Autodesk Fusion 360 part; units mm, degrees
note: some values were not read from the file. Chosen so that the rebuilt part matches the saved one: which bodies a step acts on; a direction. Set by a fixed rule: which sketch regions a step uses.
(part 3 of 5)
extrude "VL53L0X chip FL" add sketch "VL53L0X chip FL sketch" along normal blind 2.4 from surface at 101.6 separate body makes body 56 in component "ToF FL"
sketch "M2.5 screw heads FL sketch" plane through (0, 0, 0) normal (0, 0, 1) x (1, 0, 0) in component "ToF FL"
  line L0 (84.9852, 42.2659) -> (86.3446, 42.8999)
  line L1 (86.3446, 42.8999) -> (84.4428, 46.9782)
  line L2 (84.4428, 46.9782) -> (83.0834, 46.3443)
  line L3 (83.0834, 46.3443) -> (84.9852, 42.2659)
  line L4 (90.3524, 30.7558) -> (91.7119, 31.3898)
  line L5 (91.7119, 31.3898) -> (89.8101, 35.4681)
  line L6 (89.8101, 35.4681) -> (88.4506, 34.8342)
  line L7 (88.4506, 34.8342) -> (90.3524, 30.7558)
extrude "M2.5 screw heads FL" add sketch "M2.5 screw heads FL sketch" along normal blind 4.5 from surface at 110.71 separate body makes body 57 at (84.3512, 43.6254, 113.71) makes body 58 at (89.0846, 33.4748, 112.21) in component "ToF FL"
sketch "M2.5 screw shafts FL sketch" plane through (0, 0, 0) normal (0, 0, 1) x (1, 0, 0) in component "ToF FL"
  line L0 (85.8164, 44.0327) -> (91.2542, 46.5685)
  line L1 (91.2542, 46.5685) -> (90.409, 48.3811)
  line L2 (90.409, 48.3811) -> (84.9711, 45.8454)
  line L3 (84.9711, 45.8454) -> (85.8164, 44.0327)
  line L4 (91.1836, 32.5226) -> (96.6215, 35.0583)
  line L5 (96.6215, 35.0583) -> (95.7762, 36.871)
  line L6 (95.7762, 36.871) -> (90.3384, 34.3353)
  line L7 (90.3384, 34.3353) -> (91.1836, 32.5226)
extrude "M2.5 screw shafts FL" add sketch "M2.5 screw shafts FL sketch" along normal blind 2 from surface at 111.96 separate body makes body 59 at (88.8781, 46.9316, 111.96) makes body 60 at (93.9636, 36.0257, 112.6267) in component "ToF FL"
sketch "VL53L0X board FR sketch" plane through (0, 0, 0) normal (0, 0, 1) x (1, 0, 0) in component "ToF FR"
  line L0 (84.3203, -47.2411) -> (85.7704, -47.9173)
  line L1 (85.7704, -47.9173) -> (93.2845, -31.8031)
  line L2 (93.2845, -31.8031) -> (91.8344, -31.1269)
  line L3 (91.8344, -31.1269) -> (84.3203, -47.2411)
extrude "VL53L0X board FR" add sketch "VL53L0X board FR sketch" along normal blind 25.4 from surface at 90.1 separate body makes body 61 in component "ToF FR"
sketch "Board holes sketch (3)" plane through (0, 0, 0) normal (0, 0, 1) x (1, 0, 0) in component "ToF FR"
  line L0 (89.7796, -34.3505) -> (92.136, -35.4493)
  line L1 (92.136, -35.4493) -> (93.1925, -33.1836)
  line L2 (93.1925, -33.1836) -> (90.8361, -32.0848)
  line L3 (90.8361, -32.0848) -> (89.7796, -34.3505)
  line L4 (84.4123, -45.8606) -> (86.7687, -46.9594)
  line L5 (86.7687, -46.9594) -> (87.8253, -44.6937)
  line L6 (87.8253, -44.6937) -> (85.4689, -43.5949)
  line L7 (85.4689, -43.5949) -> (84.4123, -45.8606)
extrude "Board holes''" cut sketch "Board holes sketch (3)" along normal blind 2.5 from surface at 111.71 bodies 61 in component "ToF FR"
sketch "Board holes sketch (1) (3)" plane through (0, 0, 0) normal (0, 0, 1) x (1, 0, 0) in component "ToF FR"
  line L0 (89.7796, -34.3505) -> (92.136, -35.4493)
  line L1 (92.136, -35.4493) -> (93.1925, -33.1836)
  line L2 (93.1925, -33.1836) -> (90.8361, -32.0848)
  line L3 (90.8361, -32.0848) -> (89.7796, -34.3505)
  line L4 (84.4123, -45.8606) -> (86.7687, -46.9594)
  line L5 (86.7687, -46.9594) -> (87.8253, -44.6937)
  line L6 (87.8253, -44.6937) -> (85.4689, -43.5949)
  line L7 (85.4689, -43.5949) -> (84.4123, -45.8606)
extrude "Board holes (1)''" cut sketch "Board holes sketch (1) (3)" along normal blind 2.5 from surface at 91.39 bodies 61 in component "ToF FR"
sketch "QT connector FR sketch" plane through (0, 0, 0) normal (0, 0, 1) x (1, 0, 0) in component "ToF FR"
  line L0 (88.2385, -42.6244) -> (91.0027, -43.9134)
  line L1 (91.0027, -43.9134) -> (93.5807, -38.3849)
  line L2 (93.5807, -38.3849) -> (90.8164, -37.096)
  line L3 (90.8164, -37.096) -> (88.2385, -42.6244)
extrude "QT connector FR" add sketch "QT connector FR sketch" along normal blind 4.25 from surface at 110.67 separate body makes body 62 in component "ToF FR"
sketch "QT connector FR sketch (1)" plane through (0, 0, 0) normal (0, 0, 1) x (1, 0, 0) in component "ToF FR"
  line L0 (88.2385, -42.6244) -> (91.0027, -43.9134)
  line L1 (91.0027, -43.9134) -> (93.5807, -38.3849)
  line L2 (93.5807, -38.3849) -> (90.8164, -37.096)
  line L3 (90.8164, -37.096) -> (88.2385, -42.6244)
extrude "QT connector FR (1)" add sketch "QT connector FR sketch (1)" along normal blind 4.25 from surface at 90.68 separate body makes body 63 in component "ToF FR"
sketch "VL53L0X chip FR sketch" plane through (0, 0, 0) normal (0, 0, 1) x (1, 0, 0) in component "ToF FR"
  line L0 (88.5977, -41.8541) -> (89.504, -42.2767)
  line L1 (89.504, -42.2767) -> (91.3635, -38.2889)
  line L2 (91.3635, -38.2889) -> (90.4572, -37.8663)
  line L3 (90.4572, -37.8663) -> (88.5977, -41.8541)
extrude "VL53L0X chip FR" add sketch "VL53L0X chip FR sketch" along normal blind 2.4 from surface at 101.6 separate body makes body 64 in component "ToF FR"
sketch "M2.5 screw heads FR sketch" plane through (0, 0, 0) normal (0, 0, 1) x (1, 0, 0) in component "ToF FR"
  line L0 (88.4506, -34.8342) -> (89.8101, -35.4681)
  line L1 (89.8101, -35.4681) -> (91.7119, -31.3898)
  line L2 (91.7119, -31.3898) -> (90.3524, -30.7558)
  line L3 (90.3524, -30.7558) -> (88.4506, -34.8342)
  line L4 (83.0834, -46.3443) -> (84.4428, -46.9782)
  line L5 (84.4428, -46.9782) -> (86.3446, -42.8999)
  line L6 (86.3446, -42.8999) -> (84.9852, -42.2659)
  line L7 (84.9852, -42.2659) -> (83.0834, -46.3443)
extrude "M2.5 screw heads FR" add sketch "M2.5 screw heads FR sketch" along normal blind 4.5 from surface at 110.71 separate body makes body 65 at (89.7185, -32.1153, 112.21) makes body 66 at (83.7173, -44.9849, 113.71) in component "ToF FR"
sketch "M2.5 screw shafts FR sketch" plane through (0, 0, 0) normal (0, 0, 1) x (1, 0, 0) in component "ToF FR"
  line L0 (90.3384, -34.3353) -> (95.7762, -36.871)
  line L1 (95.7762, -36.871) -> (96.6215, -35.0583)
  line L2 (96.6215, -35.0583) -> (91.1836, -32.5226)
  line L3 (91.1836, -32.5226) -> (90.3384, -34.3353)
  line L4 (84.9711, -45.8454) -> (90.409, -48.3811)
  line L5 (90.409, -48.3811) -> (91.2542, -46.5685)
  line L6 (91.2542, -46.5685) -> (85.8164, -44.0327)
  line L7 (85.8164, -44.0327) -> (84.9711, -45.8454)
extrude "M2.5 screw shafts FR" add sketch "M2.5 screw shafts FR sketch" along normal blind 2 from surface at 111.96 separate body makes body 67 at (94.8088, -34.2131, 112.6267) makes body 68 at (87.3472, -45.4822, 111.96) in component "ToF FR"
sketch "VL53L0X board SFL sketch" plane through (0, 0, 0) normal (0, 0, 1) x (1, 0, 0) in component "ToF SFL"
  line L0 (77.39, 58.4) -> (77.39, 60)
  line L1 (77.39, 60) -> (59.61, 60)
  line L2 (59.61, 60) -> (59.61, 58.4)
  line L3 (59.61, 58.4) -> (77.39, 58.4)
extrude "VL53L0X board SFL" add sketch "VL53L0X board SFL sketch" along normal blind 25.4 from surface at 90.1 separate body makes body 69 in component "ToF SFL"
sketch "Board holes sketch (4)" plane through (0, 0, 0) normal (0, 0, 1) x (1, 0, 0) in component "ToF SFL"
  line L0 (63.4, 57.9) -> (63.4, 60.5)
  line L1 (63.4, 60.5) -> (60.9, 60.5)
  line L2 (60.9, 60.5) -> (60.9, 57.9)
  line L3 (60.9, 57.9) -> (63.4, 57.9)
  line L4 (76.1, 57.9) -> (76.1, 60.5)
  line L5 (76.1, 60.5) -> (73.6, 60.5)
  line L6 (73.6, 60.5) -> (73.6, 57.9)
  line L7 (73.6, 57.9) -> (76.1, 57.9)
extrude "Board holes'''" cut sketch "Board holes sketch (4)" along normal blind 2.5 from surface at 111.71 bodies 69 in component "ToF SFL"
sketch "Board holes sketch (1) (4)" plane through (0, 0, 0) normal (0, 0, 1) x (1, 0, 0) in component "ToF SFL"
  line L0 (63.4, 57.9) -> (63.4, 60.5)
  line L1 (63.4, 60.5) -> (60.9, 60.5)
  line L2 (60.9, 60.5) -> (60.9, 57.9)
  line L3 (60.9, 57.9) -> (63.4, 57.9)
  line L4 (76.1, 57.9) -> (76.1, 60.5)
  line L5 (76.1, 60.5) -> (73.6, 60.5)
  line L6 (73.6, 60.5) -> (73.6, 57.9)
  line L7 (73.6, 57.9) -> (76.1, 57.9)
extrude "Board holes (1)'''" cut sketch "Board holes sketch (1) (4)" along normal blind 2.5 from surface at 91.39 bodies 69 in component "ToF SFL"
sketch "QT connector SFL sketch" plane through (0, 0, 0) normal (0, 0, 1) x (1, 0, 0) in component "ToF SFL"
  line L0 (71.55, 60) -> (71.55, 63.05)
  line L1 (71.55, 63.05) -> (65.45, 63.05)
  line L2 (65.45, 63.05) -> (65.45, 60)
  line L3 (65.45, 60) -> (71.55, 60)
extrude "QT connector SFL" add sketch "QT connector SFL sketch" along normal blind 4.25 from surface at 110.67 separate body makes body 70 in component "ToF SFL"
sketch "QT connector SFL sketch (1)" plane through (0, 0, 0) normal (0, 0, 1) x (1, 0, 0) in component "ToF SFL"
  line L0 (71.55, 60) -> (71.55, 63.05)
  line L1 (71.55, 63.05) -> (65.45, 63.05)
  line L2 (65.45, 63.05) -> (65.45, 60)
  line L3 (65.45, 60) -> (71.55, 60)
extrude "QT connector SFL (1)" add sketch "QT connector SFL sketch (1)" along normal blind 4.25 from surface at 90.68 separate body makes body 71 in component "ToF SFL"
sketch "VL53L0X chip SFL sketch" plane through (0, 0, 0) normal (0, 0, 1) x (1, 0, 0) in component "ToF SFL"
  line L0 (70.7, 60) -> (70.7, 61)
  line L1 (70.7, 61) -> (66.3, 61)
  line L2 (66.3, 61) -> (66.3, 60)
  line L3 (66.3, 60) -> (70.7, 60)
extrude "VL53L0X chip SFL" add sketch "VL53L0X chip SFL sketch" along normal blind 2.4 from surface at 101.6 separate body makes body 72 in component "ToF SFL"
sketch "M2.5 screw heads SFL sketch" plane through (0, 0, 0) normal (0, 0, 1) x (1, 0, 0) in component "ToF SFL"
  line L0 (64.4, 56.9) -> (64.4, 58.4)
  line L1 (64.4, 58.4) -> (59.9, 58.4)
  line L2 (59.9, 58.4) -> (59.9, 56.9)
  line L3 (59.9, 56.9) -> (64.4, 56.9)
  line L4 (77.1, 56.9) -> (77.1, 58.4)
  line L5 (77.1, 58.4) -> (72.6, 58.4)
  line L6 (72.6, 58.4) -> (72.6, 56.9)
  line L7 (72.6, 56.9) -> (77.1, 56.9)
extrude "M2.5 screw heads SFL" add sketch "M2.5 screw heads SFL sketch" along normal blind 4.5 from surface at 110.71 separate body makes body 73 at (61.4, 56.9, 112.21) makes body 74 at (74.1, 56.9, 112.21) in component "ToF SFL"
sketch "M2.5 screw shafts SFL sketch" plane through (0, 0, 0) normal (0, 0, 1) x (1, 0, 0) in component "ToF SFL"
  line L0 (63.15, 58.4) -> (63.15, 64.4)
  line L1 (63.15, 64.4) -> (61.15, 64.4)
  line L2 (61.15, 64.4) -> (61.15, 58.4)
  line L3 (61.15, 58.4) -> (63.15, 58.4)
  line L4 (75.85, 58.4) -> (75.85, 64.4)
  line L5 (75.85, 64.4) -> (73.85, 64.4)
  line L6 (73.85, 64.4) -> (73.85, 58.4)
  line L7 (73.85, 58.4) -> (75.85, 58.4)
extrude "M2.5 screw shafts SFL" add sketch "M2.5 screw shafts SFL sketch" along normal blind 2 from surface at 111.96 separate body makes body 75 at (61.15, 62.4, 112.6267) makes body 76 at (73.85, 62.4, 112.6267) in component "ToF SFL"
sketch "VL53L0X board SFR sketch" plane through (0, 0, 0) normal (0, 0, 1) x (1, 0, 0) in component "ToF SFR"
  line L0 (59.61, -58.4) -> (59.61, -60)
  line L1 (59.61, -60) -> (77.39, -60)
  line L2 (77.39, -60) -> (77.39, -58.4)
  line L3 (77.39, -58.4) -> (59.61, -58.4)
extrude "VL53L0X board SFR" add sketch "VL53L0X board SFR sketch" along normal blind 25.4 from surface at 90.1 separate body makes body 77 in component "ToF SFR"
sketch "Board holes sketch (5)" plane through (0, 0, 0) normal (0, 0, 1) x (1, 0, 0) in component "ToF SFR"
  line L0 (73.6, -57.9) -> (73.6, -60.5)
  line L1 (73.6, -60.5) -> (76.1, -60.5)
  line L2 (76.1, -60.5) -> (76.1, -57.9)
  line L3 (76.1, -57.9) -> (73.6, -57.9)
  line L4 (60.9, -57.9) -> (60.9, -60.5)
  line L5 (60.9, -60.5) -> (63.4, -60.5)
  line L6 (63.4, -60.5) -> (63.4, -57.9)
  line L7 (63.4, -57.9) -> (60.9, -57.9)
extrude "Board holes''''" cut sketch "Board holes sketch (5)" along normal blind 2.5 from surface at 111.71 bodies 77 in component "ToF SFR"
sketch "Board holes sketch (1) (5)" plane through (0, 0, 0) normal (0, 0, 1) x (1, 0, 0) in component "ToF SFR"
  line L0 (73.6, -57.9) -> (73.6, -60.5)
  line L1 (73.6, -60.5) -> (76.1, -60.5)
  line L2 (76.1, -60.5) -> (76.1, -57.9)
  line L3 (76.1, -57.9) -> (73.6, -57.9)
  line L4 (60.9, -57.9) -> (60.9, -60.5)
  line L5 (60.9, -60.5) -> (63.4, -60.5)
  line L6 (63.4, -60.5) -> (63.4, -57.9)
  line L7 (63.4, -57.9) -> (60.9, -57.9)
extrude "Board holes (1)''''" cut sketch "Board holes sketch (1) (5)" along normal blind 2.5 from surface at 91.39 bodies 77 in component "ToF SFR"
sketch "QT connector SFR sketch" plane through (0, 0, 0) normal (0, 0, 1) x (1, 0, 0) in component "ToF SFR"
  line L0 (65.45, -60) -> (65.45, -63.05)
  line L1 (65.45, -63.05) -> (71.55, -63.05)
  line L2 (71.55, -63.05) -> (71.55, -60)
  line L3 (71.55, -60) -> (65.45, -60)
extrude "QT connector SFR" add sketch "QT connector SFR sketch" along normal blind 4.25 from surface at 110.67 separate body makes body 78 in component "ToF SFR"
sketch "QT connector SFR sketch (1)" plane through (0, 0, 0) normal (0, 0, 1) x (1, 0, 0) in component "ToF SFR"
  line L0 (65.45, -60) -> (65.45, -63.05)
  line L1 (65.45, -63.05) -> (71.55, -63.05)
  line L2 (71.55, -63.05) -> (71.55, -60)
  line L3 (71.55, -60) -> (65.45, -60)
extrude "QT connector SFR (1)" add sketch "QT connector SFR sketch (1)" along normal blind 4.25 from surface at 90.68 separate body makes body 79 in component "ToF SFR"
sketch "VL53L0X chip SFR sketch" plane through (0, 0, 0) normal (0, 0, 1) x (1, 0, 0) in component "ToF SFR"
  line L0 (66.3, -60) -> (66.3, -61)
  line L1 (66.3, -61) -> (70.7, -61)
  line L2 (70.7, -61) -> (70.7, -60)
  line L3 (70.7, -60) -> (66.3, -60)
extrude "VL53L0X chip SFR" add sketch "VL53L0X chip SFR sketch" along normal blind 2.4 from surface at 101.6 separate body makes body 80 in component "ToF SFR"
sketch "M2.5 screw heads SFR sketch" plane through (0, 0, 0) normal (0, 0, 1) x (1, 0, 0) in component "ToF SFR"
  line L0 (72.6, -56.9) -> (72.6, -58.4)
  line L1 (72.6, -58.4) -> (77.1, -58.4)
  line L2 (77.1, -58.4) -> (77.1, -56.9)
  line L3 (77.1, -56.9) -> (72.6, -56.9)
  line L4 (59.9, -56.9) -> (59.9, -58.4)
  line L5 (59.9, -58.4) -> (64.4, -58.4)
  line L6 (64.4, -58.4) -> (64.4, -56.9)
  line L7 (64.4, -56.9) -> (59.9, -56.9)
extrude "M2.5 screw heads SFR" add sketch "M2.5 screw heads SFR sketch" along normal blind 4.5 from surface at 110.71 separate body makes body 81 at (75.6, -56.9, 112.21) makes body 82 at (62.9, -56.9, 112.21) in component "ToF SFR"
sketch "M2.5 screw shafts SFR sketch" plane through (0, 0, 0) normal (0, 0, 1) x (1, 0, 0) in component "ToF SFR"
  line L0 (73.85, -58.4) -> (73.85, -64.4)
  line L1 (73.85, -64.4) -> (75.85, -64.4)
  line L2 (75.85, -64.4) -> (75.85, -58.4)
  line L3 (75.85, -58.4) -> (73.85, -58.4)
  line L4 (61.15, -58.4) -> (61.15, -64.4)
  line L5 (61.15, -64.4) -> (63.15, -64.4)
  line L6 (63.15, -64.4) -> (63.15, -58.4)
  line L7 (63.15, -58.4) -> (61.15, -58.4)
extrude "M2.5 screw shafts SFR" add sketch "M2.5 screw shafts SFR sketch" along normal blind 2 from surface at 111.96 separate body makes body 83 at (75.85, -62.4, 112.6267) makes body 84 at (63.15, -62.4, 112.6267) in component "ToF SFR"
sketch "VL53L0X board SRL sketch" plane through (0, 0, 0) normal (0, 0, 1) x (1, 0, 0) in component "ToF SRL"
  line L0 (-59.61, 58.4) -> (-59.61, 60)
  line L1 (-59.61, 60) -> (-77.39, 60)
  line L2 (-77.39, 60) -> (-77.39, 58.4)
  line L3 (-77.39, 58.4) -> (-59.61, 58.4)
extrude "VL53L0X board SRL" add sketch "VL53L0X board SRL sketch" along normal blind 25.4 from surface at 90.1 separate body makes body 85 in component "ToF SRL"
sketch "Board holes sketch (6)" plane through (0, 0, 0) normal (0, 0, 1) x (1, 0, 0) in component "ToF SRL"
  line L0 (-73.6, 57.9) -> (-73.6, 60.5)
  line L1 (-73.6, 60.5) -> (-76.1, 60.5)
  line L2 (-76.1, 60.5) -> (-76.1, 57.9)
  line L3 (-76.1, 57.9) -> (-73.6, 57.9)
  line L4 (-60.9, 57.9) -> (-60.9, 60.5)
  line L5 (-60.9, 60.5) -> (-63.4, 60.5)
  line L6 (-63.4, 60.5) -> (-63.4, 57.9)
  line L7 (-63.4, 57.9) -> (-60.9, 57.9)
extrude "Board holes'''''" cut sketch "Board holes sketch (6)" along normal blind 2.5 from surface at 111.71 bodies 85 in component "ToF SRL"
sketch "Board holes sketch (1) (6)" plane through (0, 0, 0) normal (0, 0, 1) x (1, 0, 0) in component "ToF SRL"
  line L0 (-73.6, 57.9) -> (-73.6, 60.5)
  line L1 (-73.6, 60.5) -> (-76.1, 60.5)
  line L2 (-76.1, 60.5) -> (-76.1, 57.9)
  line L3 (-76.1, 57.9) -> (-73.6, 57.9)
  line L4 (-60.9, 57.9) -> (-60.9, 60.5)
  line L5 (-60.9, 60.5) -> (-63.4, 60.5)
  line L6 (-63.4, 60.5) -> (-63.4, 57.9)
  line L7 (-63.4, 57.9) -> (-60.9, 57.9)
extrude "Board holes (1)'''''" cut sketch "Board holes sketch (1) (6)" along normal blind 2.5 from surface at 91.39 bodies 85 in component "ToF SRL"
sketch "QT connector SRL sketch" plane through (0, 0, 0) normal (0, 0, 1) x (1, 0, 0) in component "ToF SRL"
  line L0 (-65.45, 60) -> (-65.45, 63.05)
  line L1 (-65.45, 63.05) -> (-71.55, 63.05)
  line L2 (-71.55, 63.05) -> (-71.55, 60)
  line L3 (-71.55, 60) -> (-65.45, 60)
extrude "QT connector SRL" add sketch "QT connector SRL sketch" along normal blind 4.25 from surface at 110.67 separate body makes body 86 in component "ToF SRL"
sketch "QT connector SRL sketch (1)" plane through (0, 0, 0) normal (0, 0, 1) x (1, 0, 0) in component "ToF SRL"
  line L0 (-65.45, 60) -> (-65.45, 63.05)
  line L1 (-65.45, 63.05) -> (-71.55, 63.05)
  line L2 (-71.55, 63.05) -> (-71.55, 60)
  line L3 (-71.55, 60) -> (-65.45, 60)
extrude "QT connector SRL (1)" add sketch "QT connector SRL sketch (1)" along normal blind 4.25 from surface at 90.68 separate body makes body 87 in component "ToF SRL"
sketch "VL53L0X chip SRL sketch" plane through (0, 0, 0) normal (0, 0, 1) x (1, 0, 0) in component "ToF SRL"
  line L0 (-66.3, 60) -> (-66.3, 61)
  line L1 (-66.3, 61) -> (-70.7, 61)
  line L2 (-70.7, 61) -> (-70.7, 60)
  line L3 (-70.7, 60) -> (-66.3, 60)
extrude "VL53L0X chip SRL" add sketch "VL53L0X chip SRL sketch" along normal blind 2.4 from surface at 101.6 separate body makes body 88 in component "ToF SRL"
sketch "M2.5 screw heads SRL sketch" plane through (0, 0, 0) normal (0, 0, 1) x (1, 0, 0) in component "ToF SRL"
  line L0 (-72.6, 56.9) -> (-72.6, 58.4)
  line L1 (-72.6, 58.4) -> (-77.1, 58.4)
  line L2 (-77.1, 58.4) -> (-77.1, 56.9)
  line L3 (-77.1, 56.9) -> (-72.6, 56.9)
  line L4 (-59.9, 56.9) -> (-59.9, 58.4)
  line L5 (-59.9, 58.4) -> (-64.4, 58.4)
  line L6 (-64.4, 58.4) -> (-64.4, 56.9)
  line L7 (-64.4, 56.9) -> (-59.9, 56.9)
extrude "M2.5 screw heads SRL" add sketch "M2.5 screw heads SRL sketch" along normal blind 4.5 from surface at 110.71 separate body makes body 89 at (-75.6, 56.9, 112.21) makes body 90 at (-62.9, 56.9, 112.21) in component "ToF SRL"
sketch "M2.5 screw shafts SRL sketch" plane through (0, 0, 0) normal (0, 0, 1) x (1, 0, 0) in component "ToF SRL"
  line L0 (-73.85, 58.4) -> (-73.85, 64.4)
  line L1 (-73.85, 64.4) -> (-75.85, 64.4)
  line L2 (-75.85, 64.4) -> (-75.85, 58.4)
  line L3 (-75.85, 58.4) -> (-73.85, 58.4)
  line L4 (-61.15, 58.4) -> (-61.15, 64.4)
  line L5 (-61.15, 64.4) -> (-63.15, 64.4)
  line L6 (-63.15, 64.4) -> (-63.15, 58.4)
  line L7 (-63.15, 58.4) -> (-61.15, 58.4)
extrude "M2.5 screw shafts SRL" add sketch "M2.5 screw shafts SRL sketch" along normal blind 2 from surface at 111.96 separate body makes body 91 at (-75.85, 62.4, 112.6267) makes body 92 at (-63.15, 62.4, 112.6267) in component "ToF SRL"
sketch "VL53L0X board SRR sketch" plane through (0, 0, 0) normal (0, 0, 1) x (1, 0, 0) in component "ToF SRR"
  line L0 (-77.39, -58.4) -> (-77.39, -60)
  line L1 (-77.39, -60) -> (-59.61, -60)
  line L2 (-59.61, -60) -> (-59.61, -58.4)
  line L3 (-59.61, -58.4) -> (-77.39, -58.4)
extrude "VL53L0X board SRR" add sketch "VL53L0X board SRR sketch" along normal blind 25.4 from surface at 90.1 separate body makes body 93 in component "ToF SRR"
sketch "Board holes sketch (7)" plane through (0, 0, 0) normal (0, 0, 1) x (1, 0, 0) in component "ToF SRR"
  line L0 (-63.4, -57.9) -> (-63.4, -60.5)
  line L1 (-63.4, -60.5) -> (-60.9, -60.5)
  line L2 (-60.9, -60.5) -> (-60.9, -57.9)
  line L3 (-60.9, -57.9) -> (-63.4, -57.9)
  line L4 (-76.1, -57.9) -> (-76.1, -60.5)
  line L5 (-76.1, -60.5) -> (-73.6, -60.5)
  line L6 (-73.6, -60.5) -> (-73.6, -57.9)
  line L7 (-73.6, -57.9) -> (-76.1, -57.9)
extrude "Board holes''''''" cut sketch "Board holes sketch (7)" along normal blind 2.5 from surface at 111.71 bodies 93 in component "ToF SRR"
sketch "Board holes sketch (1) (7)" plane through (0, 0, 0) normal (0, 0, 1) x (1, 0, 0) in component "ToF SRR"
  line L0 (-63.4, -57.9) -> (-63.4, -60.5)
  line L1 (-63.4, -60.5) -> (-60.9, -60.5)
  line L2 (-60.9, -60.5) -> (-60.9, -57.9)
  line L3 (-60.9, -57.9) -> (-63.4, -57.9)
  line L4 (-76.1, -57.9) -> (-76.1, -60.5)
  line L5 (-76.1, -60.5) -> (-73.6, -60.5)
  line L6 (-73.6, -60.5) -> (-73.6, -57.9)
  line L7 (-73.6, -57.9) -> (-76.1, -57.9)
extrude "Board holes (1)''''''" cut sketch "Board holes sketch (1) (7)" along normal blind 2.5 from surface at 91.39 bodies 93 in component "ToF SRR"
sketch "QT connector SRR sketch" plane through (0, 0, 0) normal (0, 0, 1) x (1, 0, 0) in component "ToF SRR"
  line L0 (-71.55, -60) -> (-71.55, -63.05)
  line L1 (-71.55, -63.05) -> (-65.45, -63.05)
  line L2 (-65.45, -63.05) -> (-65.45, -60)
  line L3 (-65.45, -60) -> (-71.55, -60)
extrude "QT connector SRR" add sketch "QT connector SRR sketch" along normal blind 4.25 from surface at 110.67 separate body makes body 94 in component "ToF SRR"
sketch "QT connector SRR sketch (1)" plane through (0, 0, 0) normal (0, 0, 1) x (1, 0, 0) in component "ToF SRR"
  line L0 (-71.55, -60) -> (-71.55, -63.05)
  line L1 (-71.55, -63.05) -> (-65.45, -63.05)
  line L2 (-65.45, -63.05) -> (-65.45, -60)
  line L3 (-65.45, -60) -> (-71.55, -60)
extrude "QT connector SRR (1)" add sketch "QT connector SRR sketch (1)" along normal blind 4.25 from surface at 90.68 separate body makes body 95 in component "ToF SRR"
sketch "VL53L0X chip SRR sketch" plane through (0, 0, 0) normal (0, 0, 1) x (1, 0, 0) in component "ToF SRR"
  line L0 (-70.7, -60) -> (-70.7, -61)
  line L1 (-70.7, -61) -> (-66.3, -61)
  line L2 (-66.3, -61) -> (-66.3, -60)
  line L3 (-66.3, -60) -> (-70.7, -60)
extrude "VL53L0X chip SRR" add sketch "VL53L0X chip SRR sketch" along normal blind 2.4 from surface at 101.6 separate body makes body 96 in component "ToF SRR"
sketch "M2.5 screw heads SRR sketch" plane through (0, 0, 0) normal (0, 0, 1) x (1, 0, 0) in component "ToF SRR"
  line L0 (-64.4, -56.9) -> (-64.4, -58.4)
  line L1 (-64.4, -58.4) -> (-59.9, -58.4)
  line L2 (-59.9, -58.4) -> (-59.9, -56.9)
  line L3 (-59.9, -56.9) -> (-64.4, -56.9)
  line L4 (-77.1, -56.9) -> (-77.1, -58.4)
  line L5 (-77.1, -58.4) -> (-72.6, -58.4)
  line L6 (-72.6, -58.4) -> (-72.6, -56.9)
  line L7 (-72.6, -56.9) -> (-77.1, -56.9)
extrude "M2.5 screw heads SRR" add sketch "M2.5 screw heads SRR sketch" along normal blind 4.5 from surface at 110.71 separate body makes body 97 at (-61.4, -56.9, 112.21) makes body 98 at (-74.1, -56.9, 112.21) in component "ToF SRR"
sketch "M2.5 screw shafts SRR sketch" plane through (0, 0, 0) normal (0, 0, 1) x (1, 0, 0) in component "ToF SRR"
  line L0 (-63.15, -58.4) -> (-63.15, -64.4)
  line L1 (-63.15, -64.4) -> (-61.15, -64.4)
  line L2 (-61.15, -64.4) -> (-61.15, -58.4)
  line L3 (-61.15, -58.4) -> (-63.15, -58.4)
  line L4 (-75.85, -58.4) -> (-75.85, -64.4)
  line L5 (-75.85, -64.4) -> (-73.85, -64.4)
  line L6 (-73.85, -64.4) -> (-73.85, -58.4)
  line L7 (-73.85, -58.4) -> (-75.85, -58.4)
extrude "M2.5 screw shafts SRR" add sketch "M2.5 screw shafts SRR sketch" along normal blind 2 from surface at 111.96 separate body makes body 99 at (-61.15, -62.4, 112.6267) makes body 100 at (-73.85, -62.4, 112.6267) in component "ToF SRR"
sketch "VL53L0X board RL sketch" plane through (0, 0, 0) normal (0, 0, 1) x (1, 0, 0) in component "ToF RL"
  line L0 (-82.4, 44.89) -> (-84, 44.89)
  line L1 (-84, 44.89) -> (-84, 27.11)
  line L2 (-84, 27.11) -> (-82.4, 27.11)
  line L3 (-82.4, 27.11) -> (-82.4, 44.89)
extrude "VL53L0X board RL" add sketch "VL53L0X board RL sketch" along normal blind 25.4 from surface at 90.1 separate body makes body 101 in component "ToF RL"
sketch "Board holes sketch (8)" plane through (0, 0, 0) normal (0, 0, 1) x (1, 0, 0) in component "ToF RL"
  line L0 (-81.9, 30.9) -> (-84.5, 30.9)
  line L1 (-84.5, 30.9) -> (-84.5, 28.4)
  line L2 (-84.5, 28.4) -> (-81.9, 28.4)
  line L3 (-81.9, 28.4) -> (-81.9, 30.9)
  line L4 (-81.9, 43.6) -> (-84.5, 43.6)
  line L5 (-84.5, 43.6) -> (-84.5, 41.1)
  line L6 (-84.5, 41.1) -> (-81.9, 41.1)
  line L7 (-81.9, 41.1) -> (-81.9, 43.6)
extrude "Board holes'''''''" cut sketch "Board holes sketch (8)" along normal blind 2.5 from surface at 111.71 bodies 101 in component "ToF RL"
sketch "Board holes sketch (1) (8)" plane through (0, 0, 0) normal (0, 0, 1) x (1, 0, 0) in component "ToF RL"
  line L0 (-81.9, 30.9) -> (-84.5, 30.9)
  line L1 (-84.5, 30.9) -> (-84.5, 28.4)
  line L2 (-84.5, 28.4) -> (-81.9, 28.4)
  line L3 (-81.9, 28.4) -> (-81.9, 30.9)
  line L4 (-81.9, 43.6) -> (-84.5, 43.6)
  line L5 (-84.5, 43.6) -> (-84.5, 41.1)
  line L6 (-84.5, 41.1) -> (-81.9, 41.1)
  line L7 (-81.9, 41.1) -> (-81.9, 43.6)
extrude "Board holes (1)'''''''" cut sketch "Board holes sketch (1) (8)" along normal blind 2.5 from surface at 91.39 bodies 101 in component "ToF RL"
sketch "QT connector RL sketch" plane through (0, 0, 0) normal (0, 0, 1) x (1, 0, 0) in component "ToF RL"
  line L0 (-84, 39.05) -> (-87.05, 39.05)
  line L1 (-87.05, 39.05) -> (-87.05, 32.95)
  line L2 (-87.05, 32.95) -> (-84, 32.95)
  line L3 (-84, 32.95) -> (-84, 39.05)
extrude "QT connector RL" add sketch "QT connector RL sketch" along normal blind 4.25 from surface at 110.67 separate body makes body 102 in component "ToF RL"
sketch "QT connector RL sketch (1)" plane through (0, 0, 0) normal (0, 0, 1) x (1, 0, 0) in component "ToF RL"
  line L0 (-84, 39.05) -> (-87.05, 39.05)
  line L1 (-87.05, 39.05) -> (-87.05, 32.95)
  line L2 (-87.05, 32.95) -> (-84, 32.95)
  line L3 (-84, 32.95) -> (-84, 39.05)
extrude "QT connector RL (1)" add sketch "QT connector RL sketch (1)" along normal blind 4.25 from surface at 90.68 separate body makes body 103 in component "ToF RL"
sketch "VL53L0X chip RL sketch" plane through (0, 0, 0) normal (0, 0, 1) x (1, 0, 0) in component "ToF RL"
  line L0 (-84, 38.2) -> (-85, 38.2)
  line L1 (-85, 38.2) -> (-85, 33.8)
  line L2 (-85, 33.8) -> (-84, 33.8)
  line L3 (-84, 33.8) -> (-84, 38.2)
extrude "VL53L0X chip RL" add sketch "VL53L0X chip RL sketch" along normal blind 2.4 from surface at 101.6 separate body makes body 104 in component "ToF RL"
sketch "M2.5 screw heads RL sketch" plane through (0, 0, 0) normal (0, 0, 1) x (1, 0, 0) in component "ToF RL"
  line L0 (-80.9, 31.9) -> (-82.4, 31.9)
  line L1 (-82.4, 31.9) -> (-82.4, 27.4)
  line L2 (-82.4, 27.4) -> (-80.9, 27.4)
  line L3 (-80.9, 27.4) -> (-80.9, 31.9)
  line L4 (-80.9, 44.6) -> (-82.4, 44.6)
  line L5 (-82.4, 44.6) -> (-82.4, 40.1)
  line L6 (-82.4, 40.1) -> (-80.9, 40.1)
  line L7 (-80.9, 40.1) -> (-80.9, 44.6)
extrude "M2.5 screw heads RL" add sketch "M2.5 screw heads RL sketch" along normal blind 4.5 from surface at 110.71 separate body makes body 105 at (-80.9, 28.9, 112.21) makes body 106 at (-80.9, 41.6, 112.21) in component "ToF RL"
sketch "M2.5 screw shafts RL sketch" plane through (0, 0, 0) normal (0, 0, 1) x (1, 0, 0) in component "ToF RL"
  line L0 (-82.4, 30.65) -> (-88.4, 30.65)
  line L1 (-88.4, 30.65) -> (-88.4, 28.65)
  line L2 (-88.4, 28.65) -> (-82.4, 28.65)
  line L3 (-82.4, 28.65) -> (-82.4, 30.65)
  line L4 (-82.4, 43.35) -> (-88.4, 43.35)
  line L5 (-88.4, 43.35) -> (-88.4, 41.35)
  line L6 (-88.4, 41.35) -> (-82.4, 41.35)
  line L7 (-82.4, 41.35) -> (-82.4, 43.35)
extrude "M2.5 screw shafts RL" add sketch "M2.5 screw shafts RL sketch" along normal blind 2 from surface at 111.96 separate body makes body 107 at (-86.4, 28.65, 112.6267) makes body 108 at (-84.4, 42.0167, 111.96) in component "ToF RL"
sketch "VL53L0X board RR sketch" plane through (0, 0, 0) normal (0, 0, 1) x (1, 0, 0) in component "ToF RR"
  line L0 (-82.4, -27.11) -> (-84, -27.11)
  line L1 (-84, -27.11) -> (-84, -44.89)
  line L2 (-84, -44.89) -> (-82.4, -44.89)
  line L3 (-82.4, -44.89) -> (-82.4, -27.11)
extrude "VL53L0X board RR" add sketch "VL53L0X board RR sketch" along normal blind 25.4 from surface at 90.1 separate body makes body 109 in component "ToF RR"
sketch "Board holes sketch (9)" plane through (0, 0, 0) normal (0, 0, 1) x (1, 0, 0) in component "ToF RR"
  line L0 (-81.9, -41.1) -> (-84.5, -41.1)
  line L1 (-84.5, -41.1) -> (-84.5, -43.6)
  line L2 (-84.5, -43.6) -> (-81.9, -43.6)
  line L3 (-81.9, -43.6) -> (-81.9, -41.1)
  line L4 (-81.9, -28.4) -> (-84.5, -28.4)
  line L5 (-84.5, -28.4) -> (-84.5, -30.9)
  line L6 (-84.5, -30.9) -> (-81.9, -30.9)
  line L7 (-81.9, -30.9) -> (-81.9, -28.4)
extrude "Board holes''''''''" cut sketch "Board holes sketch (9)" along normal blind 2.5 from surface at 111.71 bodies 109 in component "ToF RR"
sketch "Board holes sketch (1) (9)" plane through (0, 0, 0) normal (0, 0, 1) x (1, 0, 0) in component "ToF RR"
  line L0 (-81.9, -41.1) -> (-84.5, -41.1)
  line L1 (-84.5, -41.1) -> (-84.5, -43.6)
  line L2 (-84.5, -43.6) -> (-81.9, -43.6)
  line L3 (-81.9, -43.6) -> (-81.9, -41.1)
  line L4 (-81.9, -28.4) -> (-84.5, -28.4)
  line L5 (-84.5, -28.4) -> (-84.5, -30.9)
  line L6 (-84.5, -30.9) -> (-81.9, -30.9)
  line L7 (-81.9, -30.9) -> (-81.9, -28.4)
extrude "Board holes (1)''''''''" cut sketch "Board holes sketch (1) (9)" along normal blind 2.5 from surface at 91.39 bodies 109 in component "ToF RR"
sketch "QT connector RR sketch" plane through (0, 0, 0) normal (0, 0, 1) x (1, 0, 0) in component "ToF RR"
  line L0 (-84, -32.95) -> (-87.05, -32.95)
  line L1 (-87.05, -32.95) -> (-87.05, -39.05)
  line L2 (-87.05, -39.05) -> (-84, -39.05)
  line L3 (-84, -39.05) -> (-84, -32.95)
extrude "QT connector RR" add sketch "QT connector RR sketch" along normal blind 4.25 from surface at 110.67 separate body makes body 110 in component "ToF RR"
sketch "QT connector RR sketch (1)" plane through (0, 0, 0) normal (0, 0, 1) x (1, 0, 0) in component "ToF RR"
  line L0 (-84, -32.95) -> (-87.05, -32.95)
  line L1 (-87.05, -32.95) -> (-87.05, -39.05)
  line L2 (-87.05, -39.05) -> (-84, -39.05)
  line L3 (-84, -39.05) -> (-84, -32.95)
extrude "QT connector RR (1)" add sketch "QT connector RR sketch (1)" along normal blind 4.25 from surface at 90.68 separate body makes body 111 in component "ToF RR"
sketch "VL53L0X chip RR sketch" plane through (0, 0, 0) normal (0, 0, 1) x (1, 0, 0) in component "ToF RR"
  line L0 (-84, -33.8) -> (-85, -33.8)
  line L1 (-85, -33.8) -> (-85, -38.2)
  line L2 (-85, -38.2) -> (-84, -38.2)
  line L3 (-84, -38.2) -> (-84, -33.8)
extrude "VL53L0X chip RR" add sketch "VL53L0X chip RR sketch" along normal blind 2.4 from surface at 101.6 separate body makes body 112 in component "ToF RR"
sketch "M2.5 screw heads RR sketch" plane through (0, 0, 0) normal (0, 0, 1) x (1, 0, 0) in component "ToF RR"
  line L0 (-80.9, -40.1) -> (-82.4, -40.1)
  line L1 (-82.4, -40.1) -> (-82.4, -44.6)
  line L2 (-82.4, -44.6) -> (-80.9, -44.6)
  line L3 (-80.9, -44.6) -> (-80.9, -40.1)
  line L4 (-80.9, -27.4) -> (-82.4, -27.4)
  line L5 (-82.4, -27.4) -> (-82.4, -31.9)
  line L6 (-82.4, -31.9) -> (-80.9, -31.9)
  line L7 (-80.9, -31.9) -> (-80.9, -27.4)
extrude "M2.5 screw heads RR" add sketch "M2.5 screw heads RR sketch" along normal blind 4.5 from surface at 110.71 separate body makes body 113 at (-80.9, -43.1, 112.21) makes body 114 at (-80.9, -30.4, 112.21) in component "ToF RR"
sketch "M2.5 screw shafts RR sketch" plane through (0, 0, 0) normal (0, 0, 1) x (1, 0, 0) in component "ToF RR"
  line L0 (-82.4, -41.35) -> (-88.4, -41.35)
  line L1 (-88.4, -41.35) -> (-88.4, -43.35)
  line L2 (-88.4, -43.35) -> (-82.4, -43.35)
  line L3 (-82.4, -43.35) -> (-82.4, -41.35)
  line L4 (-82.4, -28.65) -> (-88.4, -28.65)
  line L5 (-88.4, -28.65) -> (-88.4, -30.65)
  line L6 (-88.4, -30.65) -> (-82.4, -30.65)
  line L7 (-82.4, -30.65) -> (-82.4, -28.65)
extrude "M2.5 screw shafts RR" add sketch "M2.5 screw shafts RR sketch" along normal blind 2 from surface at 111.96 separate body makes body 115 at (-84.4, -42.6833, 111.96) makes body 116 at (-86.4, -30.65, 112.6267) in component "ToF RR"
sketch "OpenMV H7 Plus board L sketch" plane through (0, 0, 0) normal (0, 0, 1) x (1, 0, 0) in component "Camera L"
  line L0 (-5, -17.78) -> (39.45, -17.78)
  line L1 (39.45, -17.78) -> (39.45, 17.78)
  line L2 (39.45, 17.78) -> (-5, 17.78)
  line L3 (-5, 17.78) -> (-5, -17.78)
extrude "OpenMV H7 Plus board L" add sketch "OpenMV H7 Plus board L sketch" along normal blind 1.6 from surface at 27.4 separate body makes body 117 in component "Camera L"
sketch "Board holes sketch (10)" plane through (0, 0, 0) normal (0, 0, 1) x (1, 0, 0) in component "Camera L"
  line L0 (-3.3, -16.2) -> (-0.5, -16.2)
  line L1 (-0.5, -16.2) -> (-0.5, -13.4)
  line L2 (-0.5, -13.4) -> (-3.3, -13.4)
  line L3 (-3.3, -13.4) -> (-3.3, -16.2)
  line L4 (-3.3, 13.3) -> (-0.5, 13.3)
  line L5 (-0.5, 13.3) -> (-0.5, 16.1)
  line L6 (-0.5, 16.1) -> (-3.3, 16.1)
  line L7 (-3.3, 16.1) -> (-3.3, 13.3)
  line L8 (1.675, -16.925) -> (4.725, -16.925)
  line L9 (4.725, -16.925) -> (4.725, -13.875)
  line L10 (4.725, -13.875) -> (1.675, -13.875)
  line L11 (1.675, -13.875) -> (1.675, -16.925)
  line L12 (1.675, 13.975) -> (4.725, 13.975)
  line L13 (4.725, 13.975) -> (4.725, 17.025)
  line L14 (4.725, 17.025) -> (1.675, 17.025)
  line L15 (1.675, 17.025) -> (1.675, 13.975)
extrude "Board holes'''''''''" cut sketch "Board holes sketch (10)" along normal blind 2.6 from surface at 26.9 bodies 117 in component "Camera L"
sketch "Lens holder L sketch" plane through (0, 0, 0) normal (0, 0, 1) x (1, 0, 0) in component "Camera L"
  line L0 (-8.7, -8.7) -> (8.7, -8.7)
  line L1 (8.7, -8.7) -> (8.7, 8.7)
  line L2 (8.7, 8.7) -> (-8.7, 8.7)
  line L3 (-8.7, 8.7) -> (-8.7, -8.7)
extrude "Lens holder L" add sketch "Lens holder L sketch" along normal blind 12 from surface at 15.4 separate body makes body 118 in component "Camera L"
sketch "Lens barrel L sketch" plane through (0, 0, 0) normal (0, 0, 1) x (1, 0, 0) in component "Camera L"
  circle A0 centre (0, 0) radius 6.25
extrude "Lens barrel L" add sketch "Lens barrel L sketch" along normal blind 15.4 separate body makes body 119 in component "Camera L"
sketch "micro-SD socket L sketch" plane through (0, 0, 0) normal (0, 0, 1) x (1, 0, 0) in component "Camera L"
  line L0 (7, 0) -> (19, 0)
  line L1 (19, 0) -> (19, 14)
  line L2 (19, 14) -> (7, 14)
  line L3 (7, 14) -> (7, 0)
extrude "micro-SD socket L" add sketch "micro-SD socket L sketch" along normal blind 2 from surface at 29 separate body makes body 120 in component "Camera L"
sketch "M2.5 screw heads L sketch" plane through (0, 0, 0) normal (0, 0, 1) x (1, 0, 0) in component "Camera L"
  line L0 (-4.15, -17.05) -> (0.35, -17.05)
  line L1 (0.35, -17.05) -> (0.35, -12.55)
  line L2 (0.35, -12.55) -> (-4.15, -12.55)
  line L3 (-4.15, -12.55) -> (-4.15, -17.05)
  line L4 (-4.15, 12.45) -> (0.35, 12.45)
  line L5 (0.35, 12.45) -> (0.35, 16.95)
  line L6 (0.35, 16.95) -> (-4.15, 16.95)
  line L7 (-4.15, 16.95) -> (-4.15, 12.45)
  line L8 (0.95, -17.65) -> (5.45, -17.65)
  line L9 (5.45, -17.65) -> (5.45, -13.15)
  line L10 (5.45, -13.15) -> (0.95, -13.15)
  line L11 (0.95, -13.15) -> (0.95, -17.65)
  line L12 (0.95, 13.25) -> (5.45, 13.25)
  line L13 (5.45, 13.25) -> (5.45, 17.75)
  line L14 (5.45, 17.75) -> (0.95, 17.75)
  line L15 (0.95, 17.75) -> (0.95, 13.25)
extrude "M2.5 screw heads L" add sketch "M2.5 screw heads L sketch" along normal blind 1.5 from surface at 29 separate body makes body 121 at (2.45, -14.65, 29) makes body 122 at (-1.15, 15.45, 29) makes body 123 at (-1.15, -15.55, 29) makes body 124 at (2.45, 16.25, 29) in component "Camera L"
sketch "M2.5 screw shafts L sketch" plane through (0, 0, 0) normal (0, 0, 1) x (1, 0, 0) in component "Camera L"
  line L0 (-2.85, -15.75) -> (-0.95, -15.75)
  line L1 (-0.95, -15.75) -> (-0.95, -13.85)
  line L2 (-0.95, -13.85) -> (-2.85, -13.85)
  line L3 (-2.85, -13.85) -> (-2.85, -15.75)
  line L4 (-2.85, 13.75) -> (-0.95, 13.75)
  line L5 (-0.95, 13.75) -> (-0.95, 15.65)
  line L6 (-0.95, 15.65) -> (-2.85, 15.65)
  line L7 (-2.85, 15.65) -> (-2.85, 13.75)
  line L8 (2.25, -16.35) -> (4.15, -16.35)
  line L9 (4.15, -16.35) -> (4.15, -14.45)
  line L10 (4.15, -14.45) -> (2.25, -14.45)
  line L11 (2.25, -14.45) -> (2.25, -16.35)
  line L12 (2.25, 14.55) -> (4.15, 14.55)
  line L13 (4.15, 14.55) -> (4.15, 16.45)
  line L14 (4.15, 16.45) -> (2.25, 16.45)
  line L15 (2.25, 16.45) -> (2.25, 14.55)
extrude "M2.5 screw shafts L" add sketch "M2.5 screw shafts L sketch" along normal blind 6 from surface at 23 separate body makes body 125 at (2.25, -15.0833, 25) makes body 126 at (-1.5833, 15.65, 25) makes body 127 at (-2.85, -14.4833, 25) makes body 128 at (2.8833, 14.55, 25) in component "Camera L"
sketch "Cage frame L sketch" plane through (0, 0, 0) normal (0, 0, 1) x (1, 0, 0) in component "Camera cage L"
  line L0 (-14, -18.5) -> (14, -18.5)
  line L1 (14, -18.5) -> (14, 18.5)
  line L2 (14, 18.5) -> (-14, 18.5)
  line L3 (-14, 18.5) -> (-14, -18.5)
  line L4 (-10, -11.5) -> (10, -11.5)
  line L5 (10, -11.5) -> (10, 11.5)
  line L6 (10, 11.5) -> (-10, 11.5)
  line L7 (-10, 11.5) -> (-10, -11.5)
extrude "Cage frame L" add sketch "Cage frame L sketch" along normal blind 5 from surface at 22.4 separate body makes body 129 in component "Camera cage L"
move_body "Move1'" bodies 129 to x (1, 0, 0) y (0, 0.34202, 0.939693) z (0, -0.939693, 0.34202) at (3.0712, 87.9464, 93) in component "Camera cage L"
sketch "Cage rails L sketch" plane through (0, 0, 0) normal (0, 0, 1) x (1, 0, 0) in component "Camera cage L"
  line L0 (10, -5.5) -> (14, -5.5)
  line L1 (14, -5.5) -> (14, 5.5)
  line L2 (14, 5.5) -> (10, 5.5)
  line L3 (10, 5.5) -> (10, -5.5)
  line L4 (-14, -5.5) -> (-10, -5.5)
  line L5 (-10, -5.5) -> (-10, 5.5)
  line L6 (-10, 5.5) -> (-14, 5.5)
  line L7 (-14, 5.5) -> (-14, -5.5)
extrude "Cage rails L" add sketch "Cage rails L sketch" along normal blind 14.9 from surface at 8 separate body makes body 130 at (10, 1.8333, 12.9667) makes body 131 at (-14, 1.8333, 12.9667) in component "Camera cage L"
move_body "Move2'" bodies 130 to x (1, 0, 0) y (0, 0.34202, 0.939693) z (0, -0.939693, 0.34202) at (3.0712, 87.9464, 93) in component "Camera cage L"
move_body "Move3" bodies 131 to x (1, 0, 0) y (0, 0.34202, 0.939693) z (0, -0.939693, 0.34202) at (3.0712, 87.9464, 93) in component "Camera cage L"
combine "Combine1'" operation add target body 129 tool bodies 130 131 in component "Camera cage L"
sketch "Cage flange L sketch" plane through (0, 0, 0) normal (0, 0, 1) x (1, 0, 0) in component "Camera cage L"
  line L0 (-30, -5.5) -> (30, -5.5)
  line L1 (30, -5.5) -> (30, 5.5)
  line L2 (30, 5.5) -> (-30, 5.5)
  line L3 (-30, 5.5) -> (-30, -5.5)
extrude "Cage flange L" add sketch "Cage flange L sketch" along normal blind 3 from surface at 8 separate body makes body 132 in component "Camera cage L"
move_body "Move4" bodies 132 to x (1, 0, 0) y (0, 0.34202, 0.939693) z (0, -0.939693, 0.34202) at (3.0712, 87.9464, 93) in component "Camera cage L"
combine "Combine2'" operation add target body 129 tool bodies 132 in component "Camera cage L"
sketch "Cage barrel opening L sketch" plane through (0, 0, 0) normal (0, 0, 1) x (1, 0, 0) in component "Camera cage L"
  circle A0 centre (0, 0) radius 8.5
extrude "Cage barrel opening L" add sketch "Cage barrel opening L sketch" along normal blind 5 from surface at 7 separate body makes body 133 in component "Camera cage L"
move_body "Move5" bodies 133 to x (1, 0, 0) y (0, 0.34202, 0.939693) z (0, -0.939693, 0.34202) at (3.0712, 87.9464, 93) in component "Camera cage L"
combine "Combine3" operation cut target body 129 tool bodies 133 in component "Camera cage L"
sketch "Cage pilots L sketch" plane through (0, 0, 0) normal (0, 0, 1) x (1, 0, 0) in component "Camera cage L"
  line L0 (-2.9, -15.8) -> (-0.9, -15.8)
  line L1 (-0.9, -15.8) -> (-0.9, -13.8)
  line L2 (-0.9, -13.8) -> (-2.9, -13.8)
  line L3 (-2.9, -13.8) -> (-2.9, -15.8)
  line L4 (-2.9, 13.7) -> (-0.9, 13.7)
  line L5 (-0.9, 13.7) -> (-0.9, 15.7)
  line L6 (-0.9, 15.7) -> (-2.9, 15.7)
  line L7 (-2.9, 15.7) -> (-2.9, 13.7)
  line L8 (2.2, -16.4) -> (4.2, -16.4)
  line L9 (4.2, -16.4) -> (4.2, -14.4)
  line L10 (4.2, -14.4) -> (2.2, -14.4)
  line L11 (2.2, -14.4) -> (2.2, -16.4)
  line L12 (2.2, 14.5) -> (4.2, 14.5)
  line L13 (4.2, 14.5) -> (4.2, 16.5)
  line L14 (4.2, 16.5) -> (2.2, 16.5)
  line L15 (2.2, 16.5) -> (2.2, 14.5)
extrude "Cage pilots L" add sketch "Cage pilots L sketch" along normal blind 4.8 from surface at 22.8 separate body makes body 134 at (2.2, -15.0667, 26) makes body 135 at (-2.9, 15.0333, 26) makes body 136 at (-2.9, -14.4667, 26) makes body 137 at (2.2, 15.8333, 26) in component "Camera cage L"
move_body "Move6" bodies 134 to x (1, 0, 0) y (0, 0.34202, 0.939693) z (0, -0.939693, 0.34202) at (3.0712, 87.9464, 93) in component "Camera cage L"
move_body "Move7" bodies 135 to x (1, 0, 0) y (0, 0.34202, 0.939693) z (0, -0.939693, 0.34202) at (3.0712, 87.9464, 93) in component "Camera cage L"
move_body "Move8" bodies 136 to x (1, 0, 0) y (0, 0.34202, 0.939693) z (0, -0.939693, 0.34202) at (3.0712, 87.9464, 93) in component "Camera cage L"
move_body "Move9" bodies 137 to x (1, 0, 0) y (0, 0.34202, 0.939693) z (0, -0.939693, 0.34202) at (3.0712, 87.9464, 93) in component "Camera cage L"
combine "Combine4" operation cut target body 129 tool bodies 134 135 136 137 in component "Camera cage L"
sketch "Cage ears L sketch" plane through (0, 0, 0) normal (0, 0, 1) x (1, 0, 0) in component "Camera cage L"
  line L0 (23.0712, 80) -> (33.0712, 80)
  line L1 (33.0712, 80) -> (33.0712, 83.7036)
  line L2 (33.0712, 83.7036) -> (23.0712, 83.7036)
  line L3 (23.0712, 83.7036) -> (23.0712, 80)
  line L4 (-26.9288, 80) -> (-16.9288, 80)
  line L5 (-16.9288, 80) -> (-16.9288, 85.8769)
  line L6 (-16.9288, 85.8769) -> (-26.9288, 85.8769)
  line L7 (-26.9288, 85.8769) -> (-26.9288, 80)
extrude "Cage ears L" add sketch "Cage ears L sketch" along normal blind 10 from surface at 90 separate body makes body 138 at (29.7378, 83.7036, 93.3333) makes body 139 at (-20.2622, 85.8769, 93.3333) in component "Camera cage L"
combine "Combine5" operation add target body 129 tool bodies 138 139 in component "Camera cage L"
sketch "Cage M3 hole +1 sketch" plane through (0, 0, 0) normal (0, 0, 1) x (1, 0, 0) in component "Camera cage L"
  line L0 (26.4712, 74.7036) -> (29.6712, 74.7036)
  line L1 (29.6712, 74.7036) -> (29.6712, 83.7036)
  line L2 (29.6712, 83.7036) -> (26.4712, 83.7036)
  line L3 (26.4712, 83.7036) -> (26.4712, 74.7036)
extrude "Cage M3 hole +1" cut sketch "Cage M3 hole +1 sketch" along normal blind 3.2 from surface at 93.4 bodies 129 in component "Camera cage L"
sketch "Cage M3 hole -1 sketch" plane through (0, 0, 0) normal (0, 0, 1) x (1, 0, 0) in component "Camera cage L"
  line L0 (-23.5288, 76.8769) -> (-20.3288, 76.8769)
  line L1 (-20.3288, 76.8769) -> (-20.3288, 85.8769)
  line L2 (-20.3288, 85.8769) -> (-23.5288, 85.8769)
  line L3 (-23.5288, 85.8769) -> (-23.5288, 76.8769)
extrude "Cage M3 hole -1" cut sketch "Cage M3 hole -1 sketch" along normal blind 3.2 from surface at 93.4 bodies 129 in component "Camera cage L"
sketch "OpenMV H7 Plus board R sketch" plane through (0, 0, 0) normal (0, 0, 1) x (1, 0, 0) in component "Camera R"
  line L0 (-39.45, -17.78) -> (5, -17.78)
  line L1 (5, -17.78) -> (5, 17.78)
  line L2 (5, 17.78) -> (-39.45, 17.78)
  line L3 (-39.45, 17.78) -> (-39.45, -17.78)
extrude "OpenMV H7 Plus board R" add sketch "OpenMV H7 Plus board R sketch" along normal blind 1.6 from surface at 27.4 separate body makes body 140 in component "Camera R"
sketch "Board holes sketch (11)" plane through (0, 0, 0) normal (0, 0, 1) x (1, 0, 0) in component "Camera R"
  line L0 (0.5, -16.2) -> (3.3, -16.2)
  line L1 (3.3, -16.2) -> (3.3, -13.4)
  line L2 (3.3, -13.4) -> (0.5, -13.4)
  line L3 (0.5, -13.4) -> (0.5, -16.2)
  line L4 (0.5, 13.3) -> (3.3, 13.3)
  line L5 (3.3, 13.3) -> (3.3, 16.1)
  line L6 (3.3, 16.1) -> (0.5, 16.1)
  line L7 (0.5, 16.1) -> (0.5, 13.3)
  line L8 (-4.725, -16.925) -> (-1.675, -16.925)
  line L9 (-1.675, -16.925) -> (-1.675, -13.875)
  line L10 (-1.675, -13.875) -> (-4.725, -13.875)
  line L11 (-4.725, -13.875) -> (-4.725, -16.925)
  line L12 (-4.725, 13.975) -> (-1.675, 13.975)
  line L13 (-1.675, 13.975) -> (-1.675, 17.025)
  line L14 (-1.675, 17.025) -> (-4.725, 17.025)
  line L15 (-4.725, 17.025) -> (-4.725, 13.975)
extrude "Board holes''''''''''" cut sketch "Board holes sketch (11)" along normal blind 2.6 from surface at 26.9 bodies 140 in component "Camera R"
sketch "Lens holder R sketch" plane through (0, 0, 0) normal (0, 0, 1) x (1, 0, 0) in component "Camera R"
  line L0 (-8.7, -8.7) -> (8.7, -8.7)
  line L1 (8.7, -8.7) -> (8.7, 8.7)
  line L2 (8.7, 8.7) -> (-8.7, 8.7)
  line L3 (-8.7, 8.7) -> (-8.7, -8.7)
extrude "Lens holder R" add sketch "Lens holder R sketch" along normal blind 12 from surface at 15.4 separate body makes body 141 in component "Camera R"
sketch "Lens barrel R sketch" plane through (0, 0, 0) normal (0, 0, 1) x (1, 0, 0) in component "Camera R"
  circle A0 centre (0, 0) radius 6.25
extrude "Lens barrel R" add sketch "Lens barrel R sketch" along normal blind 15.4 separate body makes body 142 in component "Camera R"
sketch "micro-SD socket R sketch" plane through (0, 0, 0) normal (0, 0, 1) x (1, 0, 0) in component "Camera R"
  line L0 (-19, 0) -> (-7, 0)
  line L1 (-7, 0) -> (-7, 14)
  line L2 (-7, 14) -> (-19, 14)
  line L3 (-19, 14) -> (-19, 0)
extrude "micro-SD socket R" add sketch "micro-SD socket R sketch" along normal blind 2 from surface at 29 separate body makes body 143 in component "Camera R"
sketch "M2.5 screw heads R sketch" plane through (0, 0, 0) normal (0, 0, 1) x (1, 0, 0) in component "Camera R"
  line L0 (-0.35, -17.05) -> (4.15, -17.05)
  line L1 (4.15, -17.05) -> (4.15, -12.55)
  line L2 (4.15, -12.55) -> (-0.35, -12.55)
  line L3 (-0.35, -12.55) -> (-0.35, -17.05)
  line L4 (-0.35, 12.45) -> (4.15, 12.45)
  line L5 (4.15, 12.45) -> (4.15, 16.95)
  line L6 (4.15, 16.95) -> (-0.35, 16.95)
  line L7 (-0.35, 16.95) -> (-0.35, 12.45)
  line L8 (-5.45, -17.65) -> (-0.95, -17.65)
  line L9 (-0.95, -17.65) -> (-0.95, -13.15)
  line L10 (-0.95, -13.15) -> (-5.45, -13.15)
  line L11 (-5.45, -13.15) -> (-5.45, -17.65)
  line L12 (-5.45, 13.25) -> (-0.95, 13.25)
  line L13 (-0.95, 13.25) -> (-0.95, 17.75)
  line L14 (-0.95, 17.75) -> (-5.45, 17.75)
  line L15 (-5.45, 17.75) -> (-5.45, 13.25)
extrude "M2.5 screw heads R" add sketch "M2.5 screw heads R sketch" along normal blind 1.5 from surface at 29 separate body makes body 144 at (-3.95, -14.65, 29) makes body 145 at (2.65, 15.45, 29) makes body 146 at (2.65, -15.55, 29) makes body 147 at (-3.95, 16.25, 29) in component "Camera R"
sketch "M2.5 screw shafts R sketch" plane through (0, 0, 0) normal (0, 0, 1) x (1, 0, 0) in component "Camera R"
  line L0 (0.95, -15.75) -> (2.85, -15.75)
  line L1 (2.85, -15.75) -> (2.85, -13.85)
  line L2 (2.85, -13.85) -> (0.95, -13.85)
  line L3 (0.95, -13.85) -> (0.95, -15.75)
  line L4 (0.95, 13.75) -> (2.85, 13.75)
  line L5 (2.85, 13.75) -> (2.85, 15.65)
  line L6 (2.85, 15.65) -> (0.95, 15.65)
  line L7 (0.95, 15.65) -> (0.95, 13.75)
  line L8 (-4.15, -16.35) -> (-2.25, -16.35)
  line L9 (-2.25, -16.35) -> (-2.25, -14.45)
  line L10 (-2.25, -14.45) -> (-4.15, -14.45)
  line L11 (-4.15, -14.45) -> (-4.15, -16.35)
  line L12 (-4.15, 14.55) -> (-2.25, 14.55)
  line L13 (-2.25, 14.55) -> (-2.25, 16.45)
  line L14 (-2.25, 16.45) -> (-4.15, 16.45)
  line L15 (-4.15, 16.45) -> (-4.15, 14.55)
extrude "M2.5 screw shafts R" add sketch "M2.5 screw shafts R sketch" along normal blind 6 from surface at 23 separate body makes body 148 at (-4.15, -15.0833, 25) makes body 149 at (2.2167, 15.65, 25) makes body 150 at (0.95, -14.4833, 25) makes body 151 at (-2.8833, 16.45, 25) in component "Camera R"
sketch "Cage frame R sketch" plane through (0, 0, 0) normal (0, 0, 1) x (1, 0, 0) in component "Camera cage R"
  line L0 (-14, -18.5) -> (14, -18.5)
  line L1 (14, -18.5) -> (14, 18.5)
  line L2 (14, 18.5) -> (-14, 18.5)
  line L3 (-14, 18.5) -> (-14, -18.5)
  line L4 (-10, -11.5) -> (10, -11.5)
  line L5 (10, -11.5) -> (10, 11.5)
  line L6 (10, 11.5) -> (-10, 11.5)
  line L7 (-10, 11.5) -> (-10, -11.5)
extrude "Cage frame R" add sketch "Cage frame R sketch" along normal blind 5 from surface at 22.4 separate body makes body 152 in component "Camera cage R"
move_body "Move1''" bodies 152 to x (-1, 0, 0) y (0, -0.34202, 0.939693) z (0, 0.939693, 0.34202) at (3.0712, -87.9464, 93) in component "Camera cage R"
sketch "Cage rails R sketch" plane through (0, 0, 0) normal (0, 0, 1) x (1, 0, 0) in component "Camera cage R"
  line L0 (10, -5.5) -> (14, -5.5)
  line L1 (14, -5.5) -> (14, 5.5)
  line L2 (14, 5.5) -> (10, 5.5)
  line L3 (10, 5.5) -> (10, -5.5)
  line L4 (-14, -5.5) -> (-10, -5.5)
  line L5 (-10, -5.5) -> (-10, 5.5)
  line L6 (-10, 5.5) -> (-14, 5.5)
  line L7 (-14, 5.5) -> (-14, -5.5)
extrude "Cage rails R" add sketch "Cage rails R sketch" along normal blind 14.9 from surface at 8 separate body makes body 153 at (10, 1.8333, 12.9667) makes body 154 at (-14, 1.8333, 12.9667) in component "Camera cage R"
move_body "Move2''" bodies 153 to x (-1, 0, 0) y (0, -0.34202, 0.939693) z (0, 0.939693, 0.34202) at (3.0712, -87.9464, 93) in component "Camera cage R"